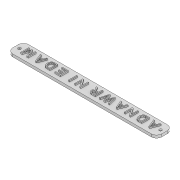
# Autodesk Inventor part: RWANDA_SIGN_MIRRORRED
Saved by Autodesk Inventor 2021 (Build 250183000, 183)
## iProperties
Created: 2021-12-15
Part Number: RWANDA_SIGN_MIRRORRED
Material: Generic
Document SubType Name: Modeling
Designer: Administrator
Density: 1 g/cm^3
Appearance: Default
Author: Administrator
Autodesk Inventor part; units mm, degrees
ref_plane "YZ Plane" through (0, 0, 0) normal (1, 0, 0) x (0, 1, 0)
ref_plane "XZ Plane" through (0, 0, 0) normal (0, 1, 0) x (-1, 0, 0)
ref_plane "XY Plane" through (0, 0, 0) normal (0, 0, 1) x (1, 0, 0)
sketch "Sketch1" plane through (0, 0, 0) normal (0, 1, 0) x (-1, 0, 0)
  line L0 (-298.1772, 27.7181) -> (276.1339, 27.7181) construction
  line L1 (276.1339, 27.7181) -> (276.1339, -22.2819) construction
  line L2 (276.1339, -22.2819) -> (-298.1772, -22.2819) construction
  line L3 (-298.1772, -22.2819) -> (-298.1772, 27.7181) construction
  line L4 (-298.2229, -2.2819) -> (-286.6985, 27.7181)
  line L5 (-286.6985, 27.7181) -> (-282.3998, 27.7181)
  line L6 (-282.3998, 27.7181) -> (-270.1437, -2.2819)
  line L7 (-270.1437, -2.2819) -> (-274.6711, -2.2819)
  line L8 (-274.6711, -2.2819) -> (-278.1467, 6.7958)
  line L9 (-278.1467, 6.7958) -> (-290.7229, 6.7958)
  line L10 (-290.7229, 6.7958) -> (-294.0156, -2.2819)
  line L11 (-294.0156, -2.2819) -> (-298.2229, -2.2819)
  line L12 (-289.5796, 10.0199) -> (-279.3815, 10.0199)
  line L13 (-279.3815, 10.0199) -> (-282.537, 18.3431)
  spline S0 degree 2 poles (-282.537, 18.3431) (-283.9546, 22.1388) (-284.6406, 24.5626) knots 0 0 0 1 1 1
  spline S1 degree 2 poles (-284.6406, 24.5626) (-285.2351, 21.6815) (-286.2641, 18.8233) knots 0 0 0 1 1 1
  line L14 (-286.2641, 18.8233) -> (-289.5796, 10.0199)
  line L15 (-255.3495, -2.2819) -> (-255.3495, 27.7181)
  line L16 (-255.3495, 27.7181) -> (-245.0141, 27.7181)
  spline S2 degree 2 poles (-245.0141, 27.7181) (-241.5156, 27.7181) (-239.6635, 27.2836) knots 0 0 0 1 1 1
  spline S3 degree 2 poles (-239.6635, 27.2836) (-237.0796, 26.6891) (-235.2732, 25.1342) knots 0 0 0 1 1 1
  spline S4 degree 2 poles (-235.2732, 25.1342) (-232.8952, 23.1449) (-230.54, 16.9025) (-230.54, 12.8781) knots 0 0 0 1 2 2 2
  spline S5 degree 2 poles (-230.54, 12.8781) (-230.54, 9.4711) (-232.1406, 4.1891) (-234.633, 0.7364) (-237.6056, -1.253) (-241.79, -2.2819) (-244.511, -2.2819) knots 0 0 0 1 2 3 4 5 5 5
  line L17 (-244.511, -2.2819) -> (-255.3495, -2.2819)
  line L18 (-251.3708, 1.2623) -> (-244.9684, 1.2623)
  spline S6 degree 2 poles (-244.9684, 1.2623) (-241.9958, 1.2623) (-238.6117, 2.3598) (-237.6284, 3.3659) knots 0 0 0 1 2 2 2
  spline S7 degree 2 poles (-237.6284, 3.3659) (-236.2107, 4.7836) (-234.633, 9.5397) (-234.633, 12.9467) knots 0 0 0 1 2 2 2
  spline S8 degree 2 poles (-234.633, 12.9467) (-234.633, 17.6571) (-237.7199, 22.7105) (-239.9379, 23.5565) knots 0 0 0 1 2 2 2
  spline S9 degree 2 poles (-239.9379, 23.5565) (-241.5385, 24.1739) (-245.0598, 24.1739) knots 0 0 0 1 1 1
  line L19 (-245.0598, 24.1739) -> (-251.3708, 24.1739)
  line L20 (-251.3708, 24.1739) -> (-251.3708, 1.2623)
  line L21 (-213.4592, -2.2819) -> (-213.4592, 27.7181)
  line L22 (-213.4592, 27.7181) -> (-209.3891, 27.7181)
  line L23 (-209.3891, 27.7181) -> (-193.6117, 4.1662)
  line L24 (-193.6117, 4.1662) -> (-193.6117, 27.7181)
  line L25 (-193.6117, 27.7181) -> (-189.8159, 27.7181)
  line L26 (-189.8159, 27.7181) -> (-189.8159, -2.2819)
  line L27 (-189.8159, -2.2819) -> (-193.886, -2.2819)
  line L28 (-193.886, -2.2819) -> (-209.6635, 21.2699)
  line L29 (-209.6635, 21.2699) -> (-209.6635, -2.2819)
  line L30 (-209.6635, -2.2819) -> (-213.4592, -2.2819)
  line L31 (-174.7931, -2.2819) -> (-163.2687, 27.7181)
  line L32 (-163.2687, 27.7181) -> (-158.9699, 27.7181)
  line L33 (-158.9699, 27.7181) -> (-146.7138, -2.2819)
  line L34 (-146.7138, -2.2819) -> (-151.2412, -2.2819)
  line L35 (-151.2412, -2.2819) -> (-154.7168, 6.7958)
  line L36 (-154.7168, 6.7958) -> (-167.2931, 6.7958)
  line L37 (-167.2931, 6.7958) -> (-170.5857, -2.2819)
  line L38 (-170.5857, -2.2819) -> (-174.7931, -2.2819)
  line L39 (-166.1498, 10.0199) -> (-155.9516, 10.0199)
  line L40 (-155.9516, 10.0199) -> (-159.1071, 18.3431)
  spline S10 degree 2 poles (-159.1071, 18.3431) (-160.5248, 22.1388) (-161.2107, 24.5626) knots 0 0 0 1 1 1
  spline S11 degree 2 poles (-161.2107, 24.5626) (-161.8052, 21.6815) (-162.8342, 18.8233) knots 0 0 0 1 1 1
  line L41 (-162.8342, 18.8233) -> (-166.1498, 10.0199)
  line L42 (-126.6833, -2.2819) -> (-134.6406, 27.7181)
  line L43 (-134.6406, 27.7181) -> (-130.5705, 27.7181)
  line L44 (-130.5705, 27.7181) -> (-125.9973, 8.0534)
  spline S12 degree 2 poles (-125.9973, 8.0534) (-125.2656, 4.9665) (-124.7168, 1.9025) knots 0 0 0 1 1 1
  spline S13 degree 2 poles (-124.7168, 1.9025) (-123.5735, 6.7272) (-123.3677, 7.4589) knots 0 0 0 1 1 1
  line L45 (-123.3677, 7.4589) -> (-117.6742, 27.7181)
  line L46 (-117.6742, 27.7181) -> (-112.8723, 27.7181)
  line L47 (-112.8723, 27.7181) -> (-108.5735, 12.5351)
  spline S14 degree 2 poles (-108.5735, 12.5351) (-106.9958, 6.8873) (-106.2412, 1.9025) knots 0 0 0 1 1 1
  spline S15 degree 2 poles (-106.2412, 1.9025) (-105.6696, 4.7608) (-104.7549, 8.4422) knots 0 0 0 1 1 1
  line L48 (-104.7549, 8.4422) -> (-100.0674, 27.7181)
  line L49 (-100.0674, 27.7181) -> (-96.0659, 27.7181)
  line L50 (-96.0659, 27.7181) -> (-104.2519, -2.2819)
  line L51 (-104.2519, -2.2819) -> (-108.1391, -2.2819)
  line L52 (-108.1391, -2.2819) -> (-114.4043, 20.5839)
  spline S16 degree 2 poles (-114.4043, 20.5839) (-115.2275, 23.4422) (-115.3647, 24.1053) knots 0 0 0 1 1 1
  spline S17 degree 2 poles (-115.3647, 24.1053) (-115.8677, 22.0473) (-116.2565, 20.5839) knots 0 0 0 1 1 1
  line L53 (-116.2565, 20.5839) -> (-122.5903, -2.2819)
  line L54 (-122.5903, -2.2819) -> (-126.6833, -2.2819)
  line L55 (-80.6543, -2.2819) -> (-80.6543, 27.7181)
  line L56 (-80.6543, 27.7181) -> (-67.3464, 27.7181)
  spline S18 degree 2 poles (-67.3464, 27.7181) (-63.3449, 27.7181) (-59.1604, 26.0946) (-56.6681, 22.0016) (-56.6681, 19.5321) knots 0 0 0 1 2 3 3 3
  spline S19 degree 2 poles (-56.6681, 19.5321) (-56.6681, 16.3309) (-60.8068, 11.9635) (-65.1056, 11.369) knots 0 0 0 1 2 2 2
  spline S20 degree 2 poles (-65.1056, 11.369) (-63.5507, 10.6144) (-62.7275, 9.8827) knots 0 0 0 1 1 1
  spline S21 degree 2 poles (-62.7275, 9.8827) (-60.9897, 8.2821) (-59.4348, 5.8812) knots 0 0 0 1 1 1
  line L57 (-59.4348, 5.8812) -> (-54.2443, -2.2819)
  line L58 (-54.2443, -2.2819) -> (-59.2062, -2.2819)
  line L59 (-59.2062, -2.2819) -> (-63.1848, 3.9605)
  spline S22 degree 2 poles (-63.1848, 3.9605) (-64.9226, 6.6586) (-67.1635, 9.5169) (-68.947, 10.683) (-69.8617, 10.9117) knots 0 0 0 1 2 3 3 3
  spline S23 degree 2 poles (-69.8617, 10.9117) (-70.5476, 11.0489) (-72.0796, 11.0489) knots 0 0 0 1 1 1
  line L60 (-72.0796, 11.0489) -> (-76.6757, 11.0489)
  line L61 (-76.6757, 11.0489) -> (-76.6757, -2.2819)
  line L62 (-76.6757, -2.2819) -> (-80.6543, -2.2819)
  line L63 (-76.6757, 14.4787) -> (-68.1467, 14.4787)
  spline S24 degree 2 poles (-68.1467, 14.4787) (-65.4257, 14.4787) (-62.3617, 15.5992) (-60.761, 18.0915) (-60.761, 19.5321) knots 0 0 0 1 2 3 3 3
  spline S25 degree 2 poles (-60.761, 19.5321) (-60.761, 21.6586) (-63.8479, 24.4025) (-67.1863, 24.4025) knots 0 0 0 1 2 2 2
  line L64 (-67.1863, 24.4025) -> (-76.6757, 24.4025)
  line L65 (-76.6757, 24.4025) -> (-76.6757, 14.4787)
  line L66 (-27.194, -2.2819) -> (-27.194, 27.7181)
  line L67 (-27.194, 27.7181) -> (-23.1238, 27.7181)
  line L68 (-23.1238, 27.7181) -> (-7.3464, 4.1662)
  line L69 (-7.3464, 4.1662) -> (-7.3464, 27.7181)
  line L70 (-7.3464, 27.7181) -> (-3.5507, 27.7181)
  line L71 (-3.5507, 27.7181) -> (-3.5507, -2.2819)
  line L72 (-3.5507, -2.2819) -> (-7.6208, -2.2819)
  line L73 (-7.6208, -2.2819) -> (-23.3982, 21.2699)
  line L74 (-23.3982, 21.2699) -> (-23.3982, -2.2819)
  line L75 (-23.3982, -2.2819) -> (-27.194, -2.2819)
  line L76 (15.428, -2.2819) -> (15.428, 27.7181)
  line L77 (15.428, 27.7181) -> (19.4066, 27.7181)
  line L78 (19.4066, 27.7181) -> (19.4066, -2.2819)
  line L79 (19.4066, -2.2819) -> (15.428, -2.2819)
  line L80 (49.7496, -2.2819) -> (49.7496, 27.7181)
  line L81 (49.7496, 27.7181) -> (71.4722, 27.7181)
  line L82 (71.4722, 27.7181) -> (71.4722, 24.1739)
  line L83 (71.4722, 24.1739) -> (53.7283, 24.1739)
  line L84 (53.7283, 24.1739) -> (53.7283, 15.0047)
  line L85 (53.7283, 15.0047) -> (70.3518, 15.0047)
  line L86 (70.3518, 15.0047) -> (70.3518, 11.4605)
  line L87 (70.3518, 11.4605) -> (53.7283, 11.4605)
  line L88 (53.7283, 11.4605) -> (53.7283, 1.2623)
  line L89 (53.7283, 1.2623) -> (72.1582, 1.2623)
  line L90 (72.1582, 1.2623) -> (72.1582, -2.2819)
  line L91 (72.1582, -2.2819) -> (49.7496, -2.2819)
  line L92 (89.2618, -2.2819) -> (89.2618, 27.7181)
  line L93 (89.2618, 27.7181) -> (99.5972, 27.7181)
  spline S26 degree 2 poles (99.5972, 27.7181) (103.0957, 27.7181) (104.9478, 27.2836) knots 0 0 0 1 1 1
  spline S27 degree 2 poles (104.9478, 27.2836) (107.5316, 26.6891) (109.338, 25.1342) knots 0 0 0 1 1 1
  spline S28 degree 2 poles (109.338, 25.1342) (111.7161, 23.1449) (114.0713, 16.9025) (114.0713, 12.8781) knots 0 0 0 1 2 2 2
  spline S29 degree 2 poles (114.0713, 12.8781) (114.0713, 9.4711) (112.4707, 4.1891) (109.9783, 0.7364) (107.0057, -1.253) (102.8213, -2.2819) (100.1002, -2.2819) knots 0 0 0 1 2 3 4 5 5 5
  line L94 (100.1002, -2.2819) -> (89.2618, -2.2819)
  line L95 (93.2405, 1.2623) -> (99.6429, 1.2623)
  spline S30 degree 2 poles (99.6429, 1.2623) (102.6155, 1.2623) (105.9996, 2.3598) (106.9829, 3.3659) knots 0 0 0 1 2 2 2
  spline S31 degree 2 poles (106.9829, 3.3659) (108.4005, 4.7836) (109.9783, 9.5397) (109.9783, 12.9467) knots 0 0 0 1 2 2 2
  spline S32 degree 2 poles (109.9783, 12.9467) (109.9783, 17.6571) (106.8914, 22.7105) (104.6734, 23.5565) knots 0 0 0 1 2 2 2
  spline S33 degree 2 poles (104.6734, 23.5565) (103.0728, 24.1739) (99.5515, 24.1739) knots 0 0 0 1 1 1
  line L96 (99.5515, 24.1739) -> (93.2405, 24.1739)
  line L97 (93.2405, 24.1739) -> (93.2405, 1.2623)
  line L98 (127.9051, -2.2819) -> (139.4295, 27.7181)
  line L99 (139.4295, 27.7181) -> (143.7283, 27.7181)
  line L100 (143.7283, 27.7181) -> (155.9844, -2.2819)
  line L101 (155.9844, -2.2819) -> (151.4569, -2.2819)
  line L102 (151.4569, -2.2819) -> (147.9813, 6.7958)
  line L103 (147.9813, 6.7958) -> (135.4051, 6.7958)
  line L104 (135.4051, 6.7958) -> (132.1124, -2.2819)
  line L105 (132.1124, -2.2819) -> (127.9051, -2.2819)
  line L106 (136.5484, 10.0199) -> (146.7466, 10.0199)
  line L107 (146.7466, 10.0199) -> (143.5911, 18.3431)
  spline S34 degree 2 poles (143.5911, 18.3431) (142.1734, 22.1388) (141.4874, 24.5626) knots 0 0 0 1 1 1
  spline S35 degree 2 poles (141.4874, 24.5626) (140.8929, 21.6815) (139.864, 18.8233) knots 0 0 0 1 1 1
  line L108 (139.864, 18.8233) -> (136.5484, 10.0199)
  line L109 (170.6643, -2.2819) -> (170.6643, 27.7181)
  line L110 (170.6643, 27.7181) -> (176.6323, 27.7181)
  line L111 (176.6323, 27.7181) -> (183.7435, 6.4757)
  spline S36 degree 2 poles (183.7435, 6.4757) (184.7268, 3.5031) (185.1841, 2.0397) knots 0 0 0 1 1 1
  spline S37 degree 2 poles (185.1841, 2.0397) (185.6871, 3.6632) (186.7847, 6.8415) knots 0 0 0 1 1 1
  line L112 (186.7847, 6.8415) -> (193.9874, 27.7181)
  line L113 (193.9874, 27.7181) -> (199.3152, 27.7181)
  line L114 (199.3152, 27.7181) -> (199.3152, -2.2819)
  line L115 (199.3152, -2.2819) -> (195.4966, -2.2819)
  line L116 (195.4966, -2.2819) -> (195.4966, 22.8248)
  line L117 (195.4966, 22.8248) -> (186.739, -2.2819)
  line L118 (186.739, -2.2819) -> (183.1719, -2.2819)
  line L119 (183.1719, -2.2819) -> (174.4829, 23.2592)
  line L120 (174.4829, 23.2592) -> (174.4829, -2.2819)
  line L121 (174.4829, -2.2819) -> (170.6643, -2.2819)
  point P0 (0, 0)
  dimension "d0" = 574.3111
  constraints: 2 other
  measures "d0" distance of L1.end L2.end
extrude "Extrusion1" add sketch "Sketch1" along normal blind 5
sketch "Sketch2" plane through (0, 0, 0) normal (0, -1, 0) x (1, 0, 0)
  line L0 (-190.2832, 27.7181) -> (-202.5393, -2.2819) projected
  line L1 (-233.7358, -17.2819) -> (326.2642, -17.2819)
  line L2 (326.2642, -17.2819) -> (326.2642, 42.7181)
  line L3 (326.2642, 42.7181) -> (-233.7358, 42.7181)
  line L4 (-233.7358, 42.7181) -> (-233.7358, -17.2819)
  line L5 (-233.7358, -17.2819) -> (326.2642, 42.7181) construction
  line L6 (326.2642, -17.2819) -> (-233.7358, 42.7181) construction
  line L7 (282.5598, -2.2819) -> (282.1898, -3.3696) projected
  line L8 (298.2229, -2.2819) -> (286.6985, 27.7181) projected
  point P0 (0, 0)
  point P1 (46.2642, 12.7181)
  point P2 (282.5598, -2.2819)
  point P3 (278.9927, -2.2819)
  dimension "d3" = 560
  dimension "d4" = 60
  dimension "d11" = 31.1965
  dimension "d12" = 15
  constraints: 12 end point, 2 midpoint, 2 parallel, 1 horizontal, 1 perpendicular, 1 other
  measures "d3" distance of L3.end L2.end
  measures "d4" distance of L2.end L1.end
  measures "d11" distance from line of L4 L0.end
  measures "d12" distance from line of point (298.223, -2.282) L1
extrude "Extrusion2" add sketch "Sketch2" along normal blind 10
fillet "Fillet2" radius 20 4 edges at (326.2642, -5, -17.2819) (-233.7358, -5, -17.2819) (-233.7358, -5, 42.7181) (326.2642, -5, 42.7181)
sketch "Sketch3" plane through (0, 0, 0) normal (0, 1, 0) x (1, 0, 0)
  line L0 (326.2642, -2.7181) -> (326.2642, -22.7181) projected
  line L1 (-233.7358, -22.7181) -> (-233.7358, -2.7181) projected
  point P0 (0, 0)
  point P1 (311.2642, -12.7181)
  point P2 (-218.7358, -12.7181)
  dimension "d14" = 15
  dimension "d15" = 15
  measures "d14" distance from line of L0 point (311.264, -12.718)
  measures "d15" distance from line of L1 point (-218.736, -12.718)
hole "Hole1" at (311.2642, 0, 12.7181) at (-218.7358, 0, 12.7181) direction (0, -1, 0) diameter 5.5 end through all countersink diameter 10.4 countersink angle 90 clearance for "Countersunk Flat Head Screw ISO 2009/7046" size "M5" standard "ISO"
body "Solid1"
